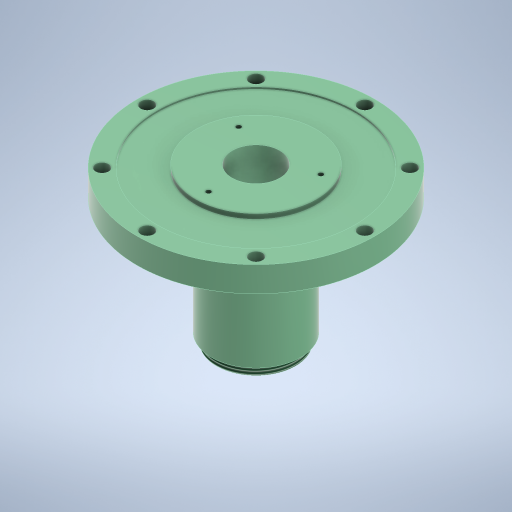
# Autodesk Inventor part: 005
Saved by Autodesk Inventor 2023 (Build 270158000, 158)
## iProperties
Created: 2021-10-30
Part Number: 005
Material: Stainless Steel, 440C
Document SubType Name: Modeling
Designer: vinicius.miguel
Density: 7.75 g/cm^3
Appearance: Smooth - Dark Sea Green
Mass: 1601.54 g
Surface Area: 443.442 cm^2
Volume: 206.65 cm^3
Author: vinicius.miguel
Autodesk Inventor part; units mm, degrees
ref_plane "YZ Plane" through (0, 0, 0) normal (1, 0, 0) x (0, 1, 0)
ref_plane "XZ Plane" through (0, 0, 0) normal (0, 1, 0) x (-1, 0, 0)
ref_plane "XY Plane" through (0, 0, 0) normal (0, 0, 1) x (1, 0, 0)
sketch "Sketch1" plane through (0, 0, 0) normal (0, 0, 1) x (1, 0, 0)
  line L0 (0, 0) -> (0, 20.5857) construction
  line L1 (12, 0) -> (12, 110)
  line L2 (12, 110) -> (30.5, 110)
  line L3 (30.5, 110) -> (30.5, 108.5)
  line L4 (30.5, 108.5) -> (60, 108.5)
  line L5 (60, 108.5) -> (60, 96.5)
  line L6 (60, 96.5) -> (22.5, 96.5)
  line L7 (22.5, 96.5) -> (22.5, 29.7)
  line L8 (22.5, 29.7) -> (14, 0)
  line L9 (14, 0) -> (12, 0)
  line L10 (30.5, 108.5) -> (30.5, 107.5)
  line L11 (30.5, 107.5) -> (50, 107.5)
  line L12 (50, 107.5) -> (50, 108.5)
  line L13 (50, 96.5) -> (50, 95.7)
  line L14 (50, 95.7) -> (60, 95.7)
  line L15 (60, 95.7) -> (60, 96.5)
  line L16 (12, 29.7) -> (15, 29.7)
  line L17 (15, 29.7) -> (15, 31.7)
  line L18 (15, 31.7) -> (20, 31.7)
  line L19 (20, 31.7) -> (20, 36.7)
  line L20 (20, 36.7) -> (22.5, 36.7)
  dimension "d36" = 110
  dimension "d38" = 24
  dimension "d39" = 28
  dimension "d40" = 45
  dimension "d41" = 1.5
  dimension "d42" = 12
  dimension "d43" = 120
  dimension "d44" = 61
  dimension "d56" = 1
  dimension "d57" = 100
  dimension "d58" = 0.8
  dimension "d77" = 30
  dimension "d78" = 40
  dimension "d79" = 2
  dimension "d80" = 5
  dimension "d83" = 2.5
  dimension "d87" = 59
  constraints: 42 end point, 14 perpendicular, 5 vertical, 4 point on line, 2 horizontal alignment, 1 parallel, 1 vertical alignment
  measures "d36" distance of L1.start L1.end
  measures "d38" diameter of L1 L0
  measures "d39" diameter of L8.end L0
  measures "d40" diameter of L7 L0
  measures "d41" distance of L2.end L3.end
  measures "d42" distance of L4.end L5.end
  measures "d43" diameter of L5 L0
  measures "d44" diameter of L3 L0
  measures "d56" distance of L3.end L10.end
  measures "d57" diameter of L12 L0
  measures "d58" distance of L13.start L13.end
  measures "d77" diameter of L17 L0
  measures "d78" diameter of L19 L0
  measures "d79" distance of L16.end L17.end
  measures "d80" distance of L18.end L19.end
  measures "d83" distance of L19.end L20.end
  measures "d87" distance from line of L14 L20.end
revolve "Revolution1" add sketch "Sketch1" angle 360 about axis through (0, 0, 0) along (0, 1, 0) contours L1 L2 L3 L10 L11 L12 L4 L5 L6 L7 L20 L19 L18 L17 L16 | L6 L15 L14 L13
sketch "Sketch3" plane through (0, 108.5, 0) normal (0, 1, 0) x (1, 0, 0)
  point P0 (0, 0)
  point P1 (55, 0)
  dimension "d45" = 55
  constraints: 1 horizontal alignment
  measures "d45" distance of point (55, 0) point (0, 0)
hole "Hole2" at (55, 108.5, 0) direction (0, -1, 0) diameter 6.6 end through all clearance for "Countersunk Flat Head Screw DIN EN ISO 2009" size "M6" standard "DIN"
pattern_circular "Circular Pattern2" count 8 over 360 about axis through (0, 102.1, 0) along (0, -1, 0) of "Hole2"
sketch "Sketch4" plane through (0, 110, 0) normal (0, 1, 0) x (1, 0, 0)
  point P0 (0, 0)
  point P1 (0, -24)
  dimension "d62" = 24
  constraints: 1 vertical alignment
  measures "d62" distance of point (0, 0) point (0, -24)
hole "Hole3" at (0, 110, 24) direction (0, -1, 0) diameter 2.459 depth 8.8 tip angle 118 thread size "M3x0.5" class "6H" standard "ISO Metric profile"
pattern_circular "Circular Pattern3" count 3 over 360 about axis through (0, 102.1, 0) along (0, -1, 0) of "Hole3"
thread "Thread4" size "M40x1.5" class "6g" standard "ISO Metric profile" length 10
body "Solid1"
